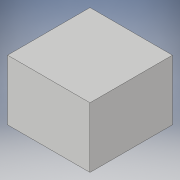
# Autodesk Inventor part: Colorimeter_Cap
Saved by Autodesk Inventor 2019 (Build 230136000, 136)
## iProperties
Created: 2019-04-03
Part Number: Colorimeter_Cap
Material: Generic
Document SubType Name: Modeling
Designer: Hansen
Density: 1 g/cm^3
Appearance: Default
Author: Hansen
Autodesk Inventor part; units mm, degrees
ref_plane "YZ Plane" through (0, 0, 0) normal (1, 0, 0) x (0, 1, 0)
ref_plane "XZ Plane" through (0, 0, 0) normal (0, 1, 0) x (-1, 0, 0)
ref_plane "XY Plane" through (0, 0, 0) normal (0, 0, 1) x (1, 0, 0)
sketch "Sketch1" plane through (0, 0, 0) normal (0, 1, 0) x (-1, 0, 0)
  line L0 (-10.25, 10.25) -> (10.25, 10.25)
  line L1 (10.25, 10.25) -> (10.25, -10.25)
  line L2 (10.25, -10.25) -> (-10.25, -10.25)
  line L3 (-10.25, -10.25) -> (-10.25, 10.25)
  line L4 (-10.25, 10.25) -> (10.25, -10.25) construction
  line L5 (10.25, 10.25) -> (-10.25, -10.25) construction
  line L6 (-8.75, 8.75) -> (8.75, 8.75)
  line L7 (8.75, 8.75) -> (8.75, -8.75)
  line L8 (8.75, -8.75) -> (-8.75, -8.75)
  line L9 (-8.75, -8.75) -> (-8.75, 8.75)
  line L10 (-8.75, 8.75) -> (8.75, -8.75) construction
  line L11 (8.75, 8.75) -> (-8.75, -8.75) construction
  point P0 (0, 0)
  dimension "d0" = 1.5
  dimension "d1" = 20.5
  constraints: 24 end point, 4 midpoint, 4 parallel, 4 perpendicular, 2 horizontal
  measures "d0" distance between parallel lines of L7 L1
  measures "d1" distance between parallel lines of L3 L1
extrude "Extrusion1" add sketch "Sketch1" along normal blind 7
sketch "Sketch2" plane through (0, 7, 0) normal (0, 1, 0) x (1, 0, 0)
  line L0 (10.25, -10.25) -> (-10.25, -10.25)
  line L1 (-10.25, -10.25) -> (-10.25, 10.25)
  line L2 (-10.25, 10.25) -> (10.25, 10.25)
  line L3 (10.25, 10.25) -> (10.25, -10.25)
  line L4 (10.25, -10.25) -> (-10.25, 10.25) construction
  line L5 (-10.25, -10.25) -> (10.25, 10.25) construction
  line L6 (7.25, -7.25) -> (-7.25, -7.25)
  line L7 (-7.25, -7.25) -> (-7.25, 7.25)
  line L8 (-7.25, 7.25) -> (7.25, 7.25)
  line L9 (7.25, 7.25) -> (7.25, -7.25)
  line L10 (7.25, -7.25) -> (-7.25, 7.25) construction
  line L11 (-7.25, -7.25) -> (7.25, 7.25) construction
  point P0 (0, 0)
  dimension "d4" = 3
  constraints: 24 end point, 4 midpoint, 4 parallel, 2 horizontal, 2 perpendicular, 1 point on line
  measures "d4" distance between parallel lines of L2 L8
extrude "Extrusion2" add sketch "Sketch2" along normal blind 5
sketch "Sketch3" plane through (0, 12, 0) normal (0, 1, 0) x (1, 0, 0)
  line L0 (-10.25, 10.25) -> (10.25, 10.25) projected
  line L1 (10.25, -10.25) -> (-10.25, -10.25)
  line L2 (-10.25, -10.25) -> (-10.25, 10.25)
  line L3 (-10.25, 10.25) -> (10.25, 10.25)
  line L4 (10.25, 10.25) -> (10.25, -10.25)
  line L5 (10.25, -10.25) -> (-10.25, 10.25) construction
  line L6 (-10.25, -10.25) -> (10.25, 10.25) construction
  point P0 (0, 0)
  constraints: 12 end point, 2 midpoint, 2 parallel, 1 horizontal, 1 perpendicular
extrude "Extrusion3" add sketch "Sketch3" along normal blind 3
body "Solid1"
